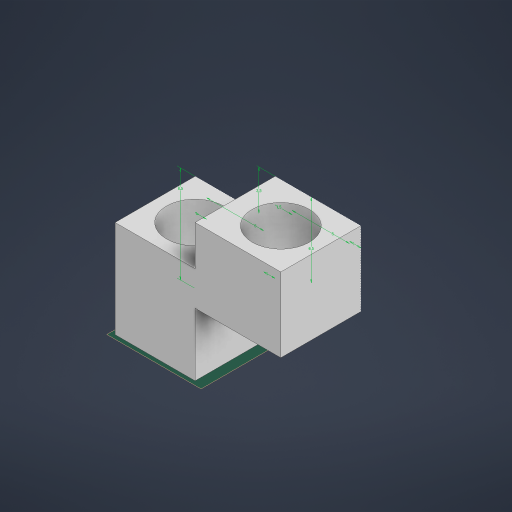
# Autodesk Inventor part: sensorholder
Saved by Autodesk Inventor 2023.4 (Build 274418000, 418)
## iProperties
Created: 2024-12-09
Part Number: sensorholder
Material: 一般
Document SubType Name: Modeling
Designer: IshiiLabHonda
Density: 1 g/cm^3
Appearance: 既定
Author: IshiiLabHonda
Autodesk Inventor part; units mm, degrees
ref_plane "YZ Plane" through (0, 0, 0) normal (1, 0, 0) x (0, 1, 0)
ref_plane "XZ Plane" through (0, 0, 0) normal (0, 1, 0) x (-1, 0, 0)
ref_plane "XY Plane" through (0, 0, 0) normal (0, 0, 1) x (1, 0, 0)
sketch "スケッチ1" plane through (0, 0, 0) normal (0, 0, 1) x (1, 0, 0)
  line L0 (-3.75, 3.25) -> (3.75, 3.25) construction
  line L1 (3.75, 3.25) -> (3.75, -3.25) construction
  line L2 (3.75, -3.25) -> (-3.75, -3.25) construction
  line L3 (-3.75, -3.25) -> (-3.75, 3.25) construction
  line L4 (0, 0) -> (0, 2.4906) construction
  line L5 (0, 0) -> (2.3218, 0) construction
  line L6 (0.25, 3.25) -> (0.25, -3.25) construction
  line L7 (-2.25, 3.25) -> (-2.25, -3.25) construction
  line L8 (2.75, 3.25) -> (2.75, -3.25) construction
  line L9 (-3.75, 3.25) -> (3.75, -3.25) construction
  line L10 (-3.75, -3.25) -> (3.75, 3.25) construction
  line L11 (-10.75, -0.25) -> (-3.75, -0.25) construction
  line L12 (-3.75, -0.25) -> (-3.75, -8.75) construction
  line L13 (-3.75, -8.75) -> (-10.75, -8.75) construction
  line L14 (-10.75, -8.75) -> (-10.75, -0.25) construction
  line L15 (-10.75, -0.25) -> (-3.75, -8.75) construction
  line L16 (-3.75, -0.25) -> (-10.75, -8.75) construction
  line L17 (-9.75, -0.25) -> (-9.75, -8.75) construction
  line L18 (-4.75, -0.25) -> (-4.75, -8.75) construction
  line L19 (-9.75, -0.25) -> (-4.75, -8.75) construction
  line L20 (-9.75, -8.75) -> (-4.75, -0.25) construction
  line L21 (-7.25, -4.5) -> (-7.25, -8.75) construction
  line L22 (-2.25, 3.25) -> (2.75, -3.25) construction
  line L23 (-2.25, -3.25) -> (2.75, 3.25) construction
  point P0 (-7.25, -4.5)
  dimension "d0" = 5
  dimension "d1" = 6.5
  dimension "d2" = 1
  dimension "d3" = 1.5
  dimension "d31" = 5
  dimension "d32" = 1
  dimension "d33" = 1
  dimension "d34" = 8.5
  dimension "d35" = 3.5
  constraints: 48 end point, 11 point on line, 9 perpendicular, 6 parallel, 5 midpoint, 1 vertical, 2 other
  measures "d0" distance between parallel lines of L7 L8
  measures "d1" distance between parallel lines of L2 L0
  measures "d2" distance between parallel lines of L1 L8
  measures "d3" distance between parallel lines of L3 L7
  measures "d31" distance between parallel lines of L18 L17
  measures "d32" distance between parallel lines of L18 L12
  measures "d33" distance between parallel lines of L14 L17
  measures "d34" distance of L13.end L11.start
  measures "d35" distance between parallel lines of L11 L0
sketch "スケッチ6" plane through (0, 0, 0) normal (0, 0, 1) x (1, 0, 0)
  line L0 (-3.75, 3.25) -> (3.75, 3.25) construction
  line L1 (3.75, 3.25) -> (3.75, -3.25) construction
  line L2 (3.75, -3.25) -> (-3.75, -3.25) construction
  line L3 (-3.75, -3.25) -> (-3.75, 3.25) construction
  line L4 (-2.25, 3.25) -> (-2.25, -3.25) construction
  line L5 (0, 0) -> (0, 2.4906) construction
  line L6 (0, 0) -> (2.3218, 0) construction
  line L7 (0.25, 3.25) -> (0.25, -3.25) construction
  line L8 (-3.75, 3.25) -> (3.75, -3.25) construction
  line L9 (-3.75, -3.25) -> (3.75, 3.25) construction
  line L10 (2.75, 3.25) -> (2.75, -3.25) construction
  line L11 (-3.75, -0.25) -> (-3.75, -8.75) construction
  line L12 (-4.75, -0.25) -> (-4.75, -8.75) construction
  line L13 (-10.75, -0.25) -> (-3.75, -0.25) construction
  line L14 (-9.75, -0.25) -> (-9.75, -8.75) construction
  line L15 (-10.75, -0.25) -> (-3.75, -8.75) construction
  line L16 (-10.75, -8.75) -> (-10.75, -0.25) construction
  line L17 (-3.75, -0.25) -> (-10.75, -8.75) construction
  line L18 (-3.75, -8.75) -> (-10.75, -8.75) construction
  line L19 (-10.75, -0.25) -> (-10.75, -8.75)
  line L20 (-3.75, -8.75) -> (-10.75, -8.75)
  line L21 (-3.75, -8.75) -> (-3.75, -3.25)
  line L22 (-3.75, -3.25) -> (3.75, -3.25)
  line L23 (3.75, -3.25) -> (3.75, 3.25)
  line L24 (3.75, 3.25) -> (-3.75, 3.25)
  line L25 (-3.75, 3.25) -> (-3.75, -0.25)
  line L26 (-10.75, -0.25) -> (-3.75, -0.25)
  line L27 (-2.25, 3.25) -> (2.75, -3.25) construction
  line L28 (-2.25, -3.25) -> (2.75, 3.25) construction
  line L29 (-7.25, -4.5) -> (-7.25, -8.75) construction
  line L30 (-9.75, -0.25) -> (-4.75, -8.75) construction
  line L31 (-9.75, -8.75) -> (-4.75, -0.25) construction
  point P0 (-7.25, -4.5)
  constraints: 16 end point, 7 perpendicular, 1 collinear
extrude "押し出し5" add sketch "スケッチ6" along normal blind 7
ref_plane "作業平面4" through (-10.75, -8.75, 0) normal (0, -1, 0) x (1, 0, 0)
sketch "スケッチ7" plane through (-10.75, -8.75, 0) normal (0, -1, 0) x (1, 0, 0)
  line L0 (7, 7) -> (14.5, 7) projected
  line L1 (14.5, 7) -> (7, 7) projected
  line L2 (7, 0) -> (7, 7) projected
  line L3 (7, 0) -> (14.5, 0) projected
  line L4 (14.5, 0) -> (14.5, 7) projected
  line L5 (7, 0) -> (7, 7) projected
  line L6 (7, 0) -> (7, 7) projected
  line L7 (14.5, 0) -> (7, 0) projected
  line L8 (14.5, 0) -> (14.5, 7) projected
  line L9 (0, 0) -> (0, 7) projected
  line L10 (0, 0) -> (7, 0) projected
  line L11 (7, 7) -> (0, 7) projected
  line L12 (0, 0) -> (0, 7) projected
  line L13 (7, 0) -> (0, 0) projected
  line L14 (0, 0) -> (7, 0) construction
  line L15 (1, 0) -> (6, 0) construction
  line L16 (1, 0) -> (6, 0) construction
  line L17 (0, 0) -> (7, 0) construction
  line L18 (7, 0) -> (0, 0) construction
  line L19 (7, 0) -> (0, 0) construction
  line L20 (7, 0) -> (14.5, 0) construction
  line L21 (14.5, 0) -> (7, 0) construction
  line L22 (10.75, 0) -> (13.0718, 0) construction
  line L23 (7, 0) -> (14.5, 0) construction
  line L24 (7, 0) -> (14.5, 0) construction
  line L25 (8.5, 0) -> (13.5, 0) construction
  line L26 (8.5, 0) -> (13.5, 0) construction
  line L27 (3.5, 0) -> (3.5, 7) construction
  line L28 (1, 0) -> (1, 7) construction
  line L29 (6, 0) -> (6, 7) construction
  line L30 (0, 7) -> (7, 7) projected
  line L31 (1, 7) -> (6, 0) construction
  line L32 (1, 0) -> (6, 7) construction
  circle A0 centre (3.5, 3.5) radius 2.5
  line L33 (8.5, 0) -> (8.5, 7) construction
  line L34 (11, 0) -> (11, 7) construction
  line L35 (13.5, 0) -> (13.5, 7) construction
  line L36 (8.5, 7) -> (13.5, 0) construction
  line L37 (8.5, 0) -> (13.5, 7) construction
  circle A1 centre (11, 3.5) radius 2.5
  point P0 (3.5, 0)
  point P1 (3.5, 0)
  point P2 (10.75, 0)
  point P3 (11, 0)
  dimension "d39" = 5
  dimension "d40" = 5
  constraints: 20 end point, 5 point on line, 3 midpoint, 3 parallel, 3 vertical, 2 centre point, 16 other
  measures "d39" diameter of A0
  measures "d40" diameter of A1
extrude "押し出し6" cut sketch "スケッチ7" against normal blind 20 contours A0 | A1
